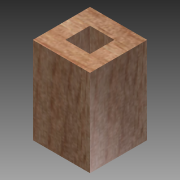
# Autodesk Inventor part: Robot-Base-Mast-Support
Saved by Autodesk Inventor 2012 (Build 160160000, 160)
## iProperties
Created: 2013-07-14
Part Number: Robot-Base-Mast-Support
Material: Wood (Birch)
Document SubType Name: Modeling
Designer: joe_000
Density: 0.55 g/cm^3
Mass: 59.9565 g
Surface Area: 203.93 cm^2
Volume: 109.012 cm^3
Author: joe_000
Autodesk Inventor part; units mm, degrees
ref_plane "YZ Plane" through (0, 0, 0) normal (1, 0, 0) x (0, 1, 0)
ref_plane "XZ Plane" through (0, 0, 0) normal (0, 1, 0) x (-1, 0, 0)
ref_plane "XY Plane" through (0, 0, 0) normal (0, 0, 1) x (1, 0, 0)
sketch "Sketch1" plane through (0, 0, 0) normal (0, 1, 0) x (-1, 0, 0)
  line L0 (0, 0) -> (-44.45, 0)
  line L1 (-44.45, 0) -> (-44.45, -44.45)
  line L2 (-44.45, -44.45) -> (0, -44.45)
  line L3 (0, -44.45) -> (0, 0)
  line L4 (-12.7, -12.7) -> (-31.75, -12.7)
  line L5 (-31.75, -12.7) -> (-31.75, -31.75)
  line L6 (-31.75, -31.75) -> (-12.7, -31.75)
  line L7 (-12.7, -31.75) -> (-12.7, -12.7)
  dimension "InnerWidth" = 19.05
  dimension "InnerWidth2" = 19.05
  dimension "Width" = 44.45
  dimension "Width2" = 44.45
  dimension "d4" = 12.7
  dimension "d5" = 12.7
  constraints: 16 end point, 4 parallel, 2 horizontal, 2 perpendicular
  measures "InnerWidth" distance of L4.end L5.end
  measures "InnerWidth2" distance of L5.end L6.end
  measures "Width" distance of L1.end L2.end
  measures "Width2" distance of L0.end L1.end
  measures "d4" distance between parallel lines of L0 L4
  measures "d5" distance between parallel lines of L3 L7
extrude "Extrusion1" add sketch "Sketch1" along normal blind 67.5875
equation "\"InnerWidth\" = MastWidth"
equation "\"InnerWidth2\" = InnerWidth"
equation "\"Width\" = MastWidth + 2 * BaseSupportThickness"
equation "\"Width2\" = Width"
equation "\"d4\" = -0.5 * InnerWidth + 0.5 * Width"
equation "\"d5\" = d4"
equation "\"d6\" = BaseSupportHeight"
equation "\"MastWidth\" = 19.05"
equation "\"BaseSupportThickness\" = 12.7"
equation "\"BaseSupportHeight\" = 67.5875"
body "Solid1"
